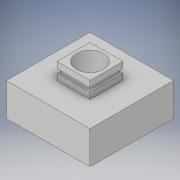
# Autodesk Inventor part: Hydraulic cylinder part 1
Saved by Autodesk Inventor 2018 (Build 220112000, 112)
## iProperties
Created: 2018-07-24
Part Number: Hydraulic cylinder part 1
Material: Generic
Document SubType Name: Modeling
Designer: BB-8
Density: 1 g/cm^3
Appearance: Default
Author: BB-8
Autodesk Inventor part; units mm, degrees
ref_plane "YZ Plane" through (0, 0, 0) normal (1, 0, 0) x (0, 1, 0)
ref_plane "XZ Plane" through (0, 0, 0) normal (0, 1, 0) x (-1, 0, 0)
ref_plane "XY Plane" through (0, 0, 0) normal (0, 0, 1) x (1, 0, 0)
sketch "Sketch2" plane through (0, 0, 0) normal (0, 1, 0) x (-1, 0, 0)
  point P0 (0, 0)
sketch "Sketch3" plane through (0, 0, 0) normal (0, 1, 0) x (-1, 0, 0)
  line L0 (0, 0) -> (76, 0)
  line L1 (76, 0) -> (76, -76)
  line L2 (76, -76) -> (0, -76)
  line L3 (0, -76) -> (0, 0)
  dimension "d1" = 76
  dimension "d2" = 76
  constraints: 8 end point, 2 parallel, 1 horizontal, 1 perpendicular
  measures "d1" distance of L1.end L2.end
  measures "d2" distance of L0.end L1.end
extrude "Extrusion1" add sketch "Sketch3" along normal blind 30
sketch "Sketch4" plane through (0, 30, 0) normal (0, 1, 0) x (1, 0, 0)
  line L0 (-76, 0) -> (0, 0) projected
  line L1 (0, 0) -> (0, 76) projected
  line L2 (-23, 23) -> (-53, 23)
  line L3 (-53, 23) -> (-53, 53)
  line L4 (-53, 53) -> (-23, 53)
  line L5 (-23, 53) -> (-23, 23)
  point P0 (-38, 38)
  dimension "d5" = 30
  dimension "d6" = 30
  constraints: 8 end point, 2 parallel, 1 horizontal, 1 perpendicular
  measures "d5" distance of L3.end L4.end
  measures "d6" distance of L2.end L3.end
extrude "Extrusion2" add sketch "Sketch4" along normal blind 15
sketch "Sketch5" plane through (-23, 30, -23) normal (1, 0, 0) x (0, 0, -1)
  line L0 (0, 0) -> (0, 15) projected
  line L1 (30, 0) -> (30, 15) projected
  line L2 (0, 5.6) -> (30, 5.6)
  line L3 (30, 5.6) -> (30, 9.4)
  line L4 (30, 9.4) -> (0, 9.4)
  line L5 (0, 9.4) -> (0, 5.6)
  point P0 (-23, -30)
  point P1 (15, 7.5)
  dimension "d9" = 3.8
  constraints: 8 end point, 2 parallel, 1 horizontal, 1 perpendicular, 1 point on line
  measures "d9" distance of L3.end L2.end
sketch "Sketch6" plane through (-23, 30, -53) normal (0, 0, -1) x (-1, 0, 0)
  line L0 (0, 0) -> (0, 15) projected
  line L1 (30, 0) -> (30, 15) projected
  line L2 (0, 5.6) -> (30, 5.6)
  line L3 (30, 5.6) -> (30, 9.4)
  line L4 (30, 9.4) -> (0, 9.4)
  line L5 (0, 9.4) -> (0, 5.6)
  point P0 (-23, -30)
  point P1 (15, 7.5)
  dimension "d10" = 3.8
  constraints: 8 end point, 2 parallel, 1 horizontal, 1 perpendicular, 1 point on line
  measures "d10" distance of L3.end L2.end
sketch "Sketch7" plane through (-53, 30, -53) normal (-1, 0, 0) x (0, 0, 1)
  line L0 (0, 0) -> (0, 15) projected
  line L1 (30, 0) -> (30, 15) projected
  line L2 (0, 5.6) -> (30, 5.6)
  line L3 (30, 5.6) -> (30, 9.4)
  line L4 (30, 9.4) -> (0, 9.4)
  line L5 (0, 9.4) -> (0, 5.6)
  point P0 (53, -30)
  point P1 (15, 7.5)
  dimension "d11" = 3.8
  constraints: 8 end point, 2 parallel, 1 horizontal, 1 perpendicular, 1 point on line
  measures "d11" distance of L3.end L2.end
sketch "Sketch8" plane through (-53, 30, -23) normal (0, 0, 1) x (1, 0, 0)
  line L0 (0, 0) -> (0, 15) projected
  line L1 (30, 0) -> (30, 15) projected
  line L2 (0, 5.6) -> (30, 5.6)
  line L3 (30, 5.6) -> (30, 9.4)
  line L4 (30, 9.4) -> (0, 9.4)
  line L5 (0, 9.4) -> (0, 5.6)
  point P0 (53, -30)
  point P1 (15, 7.5)
  dimension "d12" = 3.8
  constraints: 8 end point, 2 parallel, 1 horizontal, 1 perpendicular, 1 point on line
  measures "d12" distance of L3.end L2.end
extrude "Extrusion3" cut sketch "Sketch8" against normal blind 2
extrude "Extrusion4" cut sketch "Sketch7" against normal blind 2
extrude "Extrusion5" cut sketch "Sketch6" against normal blind 2
extrude "Extrusion6" cut sketch "Sketch5" against normal blind 2
sketch "Sketch9" plane through (0, 45, 0) normal (0, 1, 0) x (1, 0, 0)
  line L0 (-23, 53) -> (-53, 53) projected
  line L1 (-53, 23) -> (-23, 23) projected
  circle A0 centre (-38, 38) radius 12.5
  point P0 (0, 0)
  dimension "d21" = 25
  constraints: 1 centre point
  measures "d21" diameter of A0
extrude "Extrusion7" cut sketch "Sketch9" against normal blind 25
body "Solid2"
